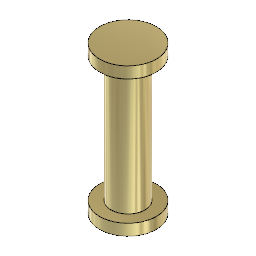
Pino_13mm_v2 (Autodesk Fusion 360 design; units mm, degrees)
Autodesk Fusion 360 part; units mm, degrees
sketch "Sketch1" plane through (0, 0, 0) normal (1, 0, 0) x (0, 1, 0)
  line L0 (10, 0.1993) -> (10, 13.1993)
  line L1 (10, 13.1993) -> (7.5, 13.1993)
  line L2 (7.5, 13.1993) -> (7.5, 12.1993)
  line L3 (7.5, 12.1993) -> (8.5, 12.1993)
  line L4 (8.5, 12.1993) -> (8.5, 1.1993)
  line L5 (8.5, 1.1993) -> (7.5, 1.1993)
  line L6 (7.5, 1.1993) -> (7.5, 0.1993)
  line L7 (7.5, 0.1993) -> (10, 0.1993)
  dimension "d1" = 13
  dimension "d2" = 1.5
  dimension "d3" = 1
  dimension "d4" = 2.5
  dimension "d5" = 1
  dimension "d6" = 2.5
  constraint vertical L0
  constraint perpendicular L0 L1
  constraint perpendicular L1 L2
  constraint perpendicular L2 L3
  constraint perpendicular L3 L4
  constraint perpendicular L4 L5
  constraint perpendicular L5 L6
  constraint perpendicular L0 L7
  measures "d1" distance of L0.start L0.end
  measures "d2" distance of L0 L4
  measures "d3" distance of L1.end L2.end
  measures "d4" distance of L0.end L1.end
  measures "d5" distance of L5.end L6.end
  measures "d6" distance of L0.start L6.end
revolve "Revolve1" add sketch "Sketch1" angle 360 about axis through (0, 10, 0.1993) along (0, 0, 1) in component "Component"
component "Component" placed x (1, 0, 0) y (0, 1, 0) z (0, 0, 1) at (0, 0, 0)
